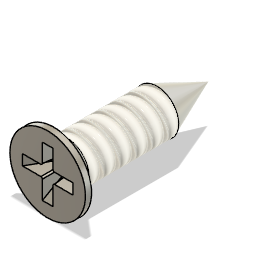
2f7473f9-b099-412f-9152-2018551abb9a (Autodesk Fusion 360 design; units mm, degrees)
description: Tipo II - Parafuso Phillips autorroscante de cabeça chata escareada a 100° ASME B18.6.4 6-20 x 0.5 Tipo AB
part number: 100CRFCHTSTATII ASME B18.6.4 - #6-20 x 1/2 Aço grau 2 Liso
Autodesk Fusion 360 part; units mm, degrees
sketch "Sketch1" plane through (0, 0, 0) normal (0, 1, 0) x (1, 0, 0)
  line L0 (0, -2.9946) -> (-2.9845, -2.9946)
  line L1 (-2.9845, -2.9946) -> (-2.9845, -2.5043)
  line L2 (-2.9845, -2.5043) -> (-1.7526, -1.4706)
  line L3 (-1.7526, -1.4706) -> (-1.7526, 9.7054)
  line L4 (0, 9.7054) -> (0, -2.9946)
  line L5 (-1.7526, 9.7054) -> (0, 9.7054)
  dimension "d9" = 3.5052
  dimension "d11" = 5.969
  dimension "d75" = 1.524
  dimension "d107" = 12.7
  dimension "d116" = 50
  constraint perpendicular L0 L1
  constraint vertical L3
  constraint perpendicular L0 L4
  constraint collinear origin L0.start L4.start
  constraint horizontal L0
  constraint horizontal L5
  constraint coincident origin L2
  measures "d75" distance of L0 L2.end
  measures "d107" distance of L0 L5
  measures "d116" angle of L2 L4
revolve "Revolve1" add sketch "Sketch1" angle 360 about axis through (0, 0, -9.7054) along (0, 0, 1) makes body 1
sketch "Sketch2" plane through (0, 0, 2.9946) normal (0, 0, 1) x (1, 0, 0)
  line L0 (-0.4191, 0.4191) -> (-1.9939, 0.4191)
  line L1 (-1.9939, 0.4191) -> (-1.9939, -0.4191)
  line L2 (-0.4191, -0.4191) -> (-1.9939, -0.4191)
  line L3 (-0.4191, -0.4191) -> (-0.4191, -1.9939)
  line L4 (-0.4191, -1.9939) -> (0.4191, -1.9939)
  line L5 (0.4191, -0.4191) -> (0.4191, -1.9939)
  line L6 (0.4191, -0.4191) -> (1.9939, -0.4191)
  line L7 (1.9939, -0.4191) -> (1.9939, 0.4191)
  line L8 (0.4191, 0.4191) -> (1.9939, 0.4191)
  line L9 (0.4191, 0.4191) -> (0.4191, 1.9939)
  line L10 (0.4191, 1.9939) -> (-0.4191, 1.9939)
  line L11 (-0.4191, 0.4191) -> (-0.4191, 1.9939)
  dimension "d111" = 360
  dimension "d113" = 3.9878
  dimension "d117" = 0.8382
  constraint vertical L0.start L2.start
  constraint horizontal L0
  constraint coincident L8.start L9.start
  constraint perpendicular L7 L8
  measures "d113" distance of L1 L7.end
  measures "d117" distance of L0 L2
extrude "Extrude1" add sketch "Sketch2" against normal blind 2.1844 draft -4 separate body makes body 2
draft "Draft2" angle -30 neutral plane through (0, 0, 2.9946) pull (0, 0, 1) 4 faces at (-1.943, -0.0888, 2.2665) (0.0888, -1.943, 2.2665) (1.943, 0.0888, 2.2665) (-0.0888, 1.943, 2.2665) on bodies 2
fillet "Fillet3" radius 0.1196 4 edges at (-0.3427, -0.3427, 1.9024) (-0.3427, 0.3427, 1.9024) (0.3427, 0.3427, 1.9024) (0.3427, -0.3427, 1.9024) on bodies 2
combine "Combine1" operation cut target body 1 tool bodies 2
thread "Thread1" "Inch Tapping Threads 0.138 6-20 6-20 2B" major diameter 3.4417 minor diameter 2.5781 pitch 1.27 angle 60 resizes the face on face at (-1.7504, 0.0874, -2.2547) on bodies 1
sketch "Sketch6" plane through (0, 0, 0) normal (0, 1, 0) x (1, 0, 0)
  line L0 (0, 9.7054) -> (-1.7877, 9.7054)
  line L1 (-1.7877, 9.7054) -> (-1.7877, 5.4742)
  line L2 (-1.7877, 5.4742) -> (0, 9.7054)
  line L3 (0, 9.7054) -> (0, -2.9946)
  line L4 (-1.7877, 9.7054) -> (0, 9.7054)
  dimension "d108" = 1.7877
  dimension "d109" = 4.2312
  constraint perpendicular L0 L1
  constraint coincident L0.start L2.end
  measures "d108" distance of L1 L3
  measures "d109" distance of L1.end L4
revolve "Revolve3" cut sketch "Sketch6" angle 360 about axis through (0, 0, 1.75) along (0, 0, 1) bodies 1
equation "d9 = adsk_nomdia"
equation "d11 = adsk_headdia"
equation "adsk_headang = 100.00 deg"
equation "d31 = -adsk_phildepth"
equation "adsk_nomlen = 0.50 in"
equation "adsk_headh = 0.06 in"
equation "adsk_headdia = 0.235 in"
equation "adsk_nomdia = 0.138 in"
equation "adsk_phildia = 0.157 in"
equation "adsk_philwidth = 0.033 in"
equation "adsk_phildepth = 0.086 in"
equation "adsk_startlen = 0.166581 in"
equation "d75 = adsk_headh"
equation "d97 = ( adsk_nomdia / 2 ) * tan(90 deg - adsk_headang / 2) + adsk_headh"
equation "d107 = adsk_nomlen"
equation "d108 = adsk_nomdia * 0.51"
equation "d109 = adsk_startlen"
equation "d113 = adsk_phildia"
equation "d115 = adsk_phildia * 0.03"
equation "d116 = adsk_headang * 0.5"
equation "d117 = adsk_philwidth"
